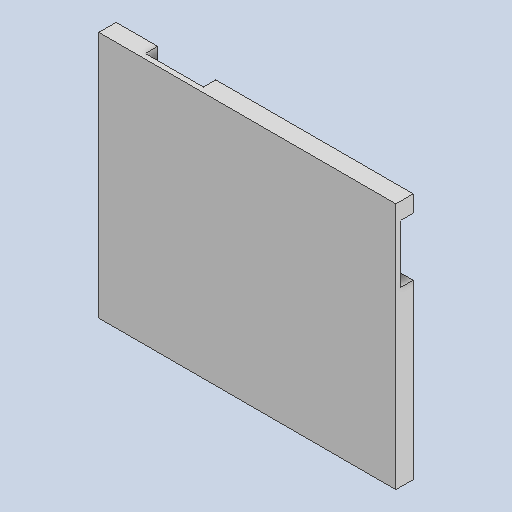
# Autodesk Inventor part: CableHolder
Saved by Autodesk Inventor 2024 (Build 280153000, 153)
## iProperties
Created: 2023-08-07
Part Number: CableHolder
Material: Generisch
Document SubType Name: Modeling
Designer: aewalder
Density: 1 g/cm^3
Appearance: Vorgabe
Author: aewalder
Autodesk Inventor part; units mm, degrees
ref_plane "YZ Plane" through (0, 0, 0) normal (1, 0, 0) x (0, 1, 0)
ref_plane "XZ Plane" through (0, 0, 0) normal (0, 1, 0) x (-1, 0, 0)
ref_plane "XY Plane" through (0, 0, 0) normal (0, 0, 1) x (1, 0, 0)
sketch "Sketch1" plane through (0, 0, 0) normal (0, 0, 1) x (1, 0, 0)
  line L0 (30, 25) -> (-30, 25) projected
  line L1 (-30, -25) -> (-30, 25) projected
  line L2 (-30, -25) -> (30, -25) projected
  line L3 (30, 25) -> (30, -25) projected
  line L4 (21.9198, 18.925) -> (23.3698, 18.925) projected
  line L5 (23.3698, 18.925) -> (23.3698, 12.575) projected
  line L6 (23.3698, 12.575) -> (21.9198, 12.575) projected
  line L7 (21.9198, 12.575) -> (21.9198, 9.885) projected
  line L8 (21.9198, 9.885) -> (-2.18, 9.885) projected
  line L9 (-2.18, 9.885) -> (-2.18, 21.615) projected
  line L10 (-2.18, 21.615) -> (21.9198, 21.615) projected
  line L11 (21.9198, 21.615) -> (21.9198, 18.925) projected
  line L12 (-12.575, 23.3698) -> (-12.575, 21.9198) projected
  line L13 (-12.575, 21.9198) -> (-9.885, 21.9198) projected
  line L14 (-9.885, 21.9198) -> (-9.885, -2.18) projected
  line L15 (-9.885, -2.18) -> (-21.615, -2.18) projected
  line L16 (-21.615, -2.18) -> (-21.615, 21.9198) projected
  line L17 (-21.615, 21.9198) -> (-18.925, 21.9198) projected
  line L18 (-18.925, 21.9198) -> (-18.925, 23.3698) projected
  line L19 (-18.925, 23.3698) -> (-12.575, 23.3698) projected
  line L20 (-23.3698, -12.575) -> (-21.9198, -12.575) projected
  line L21 (-21.9198, -12.575) -> (-21.9198, -9.885) projected
  line L22 (-21.9198, -9.885) -> (2.18, -9.885) projected
  line L23 (2.18, -9.885) -> (2.18, -21.615) projected
  line L24 (2.18, -21.615) -> (-21.9198, -21.615) projected
  line L25 (-21.9198, -21.615) -> (-21.9198, -18.925) projected
  line L26 (-21.9198, -18.925) -> (-23.3698, -18.925) projected
  line L27 (-23.3698, -18.925) -> (-23.3698, -12.575) projected
  line L28 (12.575, -23.3698) -> (12.575, -21.9198) projected
  line L29 (12.575, -21.9198) -> (9.885, -21.9198) projected
  line L30 (9.885, -21.9198) -> (9.885, 2.18) projected
  line L31 (9.885, 2.18) -> (21.615, 2.18) projected
  line L32 (21.615, 2.18) -> (21.615, -21.9198) projected
  line L33 (21.615, -21.9198) -> (18.925, -21.9198) projected
  line L34 (18.925, -21.9198) -> (18.925, -23.3698) projected
  line L35 (18.925, -23.3698) -> (12.575, -23.3698) projected
  line L36 (9.885, -21.9198) -> (9.885, -25)
  line L37 (21.615, -21.9198) -> (21.615, -25)
  line L38 (-21.9198, -21.615) -> (-30, -21.615)
  line L39 (-21.9198, -9.885) -> (-30, -9.885)
  line L40 (-21.615, 21.9198) -> (-21.615, 25)
  line L41 (-9.885, 21.9198) -> (-9.885, 25)
  line L42 (21.9198, 9.885) -> (30, 9.885)
  line L43 (21.9198, 21.615) -> (30, 21.615)
  point P0 (0, 0)
  constraints: 16 end point, 8 point on line, 7 perpendicular, 1 vertical
extrude "Extrusion1" add sketch "Sketch1" along normal blind 2.5 contours L3 L43 L10 L9 L8 L42 L2 L37 L32 L31 L30 L36 L1 L38 L24 L23 L22 L39 L0 L40 L16 L15 L14 L41
sketch "Sketch2" plane through (0, 0, 2.5) normal (0, 0, 1) x (1, 0, 0)
  line L0 (-21.615, 25) -> (-30, 25) projected
  line L1 (30, -25) -> (30, 9.885) projected
  line L2 (-30, 25) -> (30, 25)
  line L3 (30, 25) -> (30, -25)
  line L4 (30, -25) -> (-30, -25)
  line L5 (-30, -25) -> (-30, 25)
  point P0 (0, 0)
  constraints: 8 end point, 2 parallel, 1 horizontal, 1 perpendicular
extrude "Extrusion2" add sketch "Sketch2" along normal blind 1
body "Solid1"
